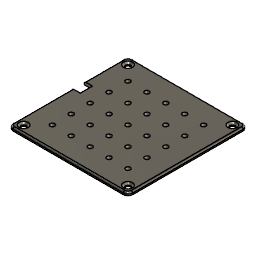
Box ESP32+CC1101 (Autodesk Fusion 360 design; units mm, degrees)
Autodesk Fusion 360 part; units mm, degrees
sketch "Base" plane through (0, 0, 0) normal (0, 0, 1) x (1, 0, 0)
  line L0 (-80.1103, 32.3186) -> (-1.1103, 32.3186)
  line L1 (-1.1103, 32.3186) -> (-1.1103, 111.3186)
  line L2 (-1.1103, 111.3186) -> (-80.1103, 111.3186)
  line L3 (-80.1103, 111.3186) -> (-80.1103, 32.3186)
  line L4 (-78.1103, 34.3186) -> (-3.1103, 34.3186)
  line L5 (-3.1103, 34.3186) -> (-3.1103, 109.3186)
  line L6 (-3.1103, 109.3186) -> (-78.1103, 109.3186)
  line L7 (-78.1103, 109.3186) -> (-78.1103, 34.3186)
  circle A0 centre (-75.1103, 106.3186) radius 5
  circle A1 centre (-6.1103, 106.3186) radius 5
  circle A2 centre (-6.1103, 37.3186) radius 5
  circle A3 centre (-75.1103, 37.3186) radius 5
  circle A4 centre (-70.6103, 106.3186) radius 2.5
  circle A5 centre (-10.6103, 106.3186) radius 2.5
  circle A6 centre (-70.6103, 48.3186) radius 2.5
  circle A7 centre (-10.6103, 48.3186) radius 2.5
  line L8 (-40.6103, 111.3186) -> (-40.6103, 44.5511) construction
  point P0 (-6.1103, 106.3186)
  point P1 (-75.1103, 106.3186)
  point P2 (-75.1103, 37.3186)
  point P3 (-6.1103, 37.3186)
  point P4 (-70.6103, 106.3186)
  point P5 (-10.6103, 106.3186)
  point P6 (-70.6103, 48.3186)
  point P7 (-10.6103, 48.3186)
  dimension "d206" = 79
  dimension "d207" = 79
  dimension "d209" = 5
  dimension "d211" = 5
  dimension "d212" = 5
  dimension "d213" = 5
  dimension "d272" = 60
  dimension "d273" = 7.5
  dimension "d276" = 3
  dimension "d278" = 60
  dimension "d279" = 7.5
  dimension "d280" = 58
  dimension "d281" = 5
  dimension "d282" = 5
  dimension "d283" = 5
  dimension "d284" = 5
  constraint horizontal L0
  constraint vertical L1
  constraint horizontal L2
  constraint vertical L3
  constraint tangent L2 A0
  constraint tangent L3 A0
  constraint tangent L2 A1
  constraint tangent L1 A1
  constraint tangent L1 A2
  constraint tangent L0 A2
  constraint tangent L3 A3
  constraint tangent L0 A3
  constraint coincident P0 A1.centre
  constraint coincident P1 A0.centre
  constraint coincident P2 A3.centre
  constraint coincident P3 A2.centre
  constraint coincident P4 A4.centre
  constraint coincident P5 A5.centre
  constraint coincident P6 A6.centre
  constraint coincident P7 A7.centre
  constraint midpoint L2 L8.start
  constraint perpendicular L6 L8
  measures "d206" distance of L0.start L0.end
  measures "d207" distance of L0.start L2.end
  measures "d209" radius of A0
  measures "d211" radius of A1
  measures "d212" radius of A2
  measures "d213" radius of A3
  measures "d272" distance of P4 P5
  measures "d273" distance of L7 P4
  measures "d276" distance of L6 P4
  measures "d278" distance of P6 P7
  measures "d279" distance of L7 P6
  measures "d280" distance of P4 P6
  measures "d281" diameter of A4
  measures "d282" diameter of A5
  measures "d283" diameter of A6
  measures "d284" diameter of A7
extrude "Extrude3" add sketch "Base" along normal blind 52 contours L0 L3 A3 | L0 L4 A2 A3 | L4 L7 A3 | L3 L7 A0 A3 | L0 L1 A2 | L4 L5 A2 | L4 L7 A3 | L2 L3 A0 | L6 L7 A0 | L4 L5 A2 | L1 L5 A1 A2 | L2 L6 A0 A1 | L6 L7 A0 A4 | L1 L2 A1 | L5 L6 A1 | A0 A4 | L5 L6 A1 A5 | A1 A5 picked at (-71.1053, 106.7133) picked at (-10.101, 106.3186) makes body 1
extrude "Extrude4" add sketch "Base" along normal blind 2 contours L4 L5 L6 L7 A0 A1 A2 A3 A4 A5 | A0 A4 | A1 A5 | A6 | A7 picked at (-69.4945, 106.7801) picked at (-11.7677, 106.3186) bodies 1
fillet "Fillet1" radius 3 4 edges at (-80.1103, 32.3186, 26) (-1.1103, 32.3186, 26) (-1.1103, 111.3186, 26) (-80.1103, 111.3186, 26) on bodies 1
sketch "Lid" plane through (0, 0, 52) normal (0, 0, 1) x (-1, 0, 0)
  arc A0 (77.1103, -111.3186) -> (80.1103, -108.3186) centre (77.1103, -108.3186) ccw
  line L0 (80.1103, -108.3186) -> (80.1103, -35.3186)
  arc A1 (80.1103, -35.3186) -> (77.1103, -32.3186) centre (77.1103, -35.3186) ccw
  line L1 (77.1103, -32.3186) -> (4.1103, -32.3186)
  arc A2 (4.1103, -32.3186) -> (1.1103, -35.3186) centre (4.1103, -35.3186) ccw
  line L2 (1.1103, -35.3186) -> (1.1103, -108.3186)
  arc A3 (1.1103, -108.3186) -> (4.1103, -111.3186) centre (4.1103, -108.3186) ccw
  line L3 (4.1103, -111.3186) -> (77.1103, -111.3186)
  line L4 (3.1103, -102.3186) -> (3.1103, -41.3186)
  arc A4 (3.1103, -41.3186) -> (10.1103, -34.3186) centre (6.1103, -37.3186) ccw
  line L5 (10.1103, -34.3186) -> (71.1103, -34.3186)
  arc A5 (71.1103, -34.3186) -> (78.1103, -41.3186) centre (75.1103, -37.3186) ccw
  line L6 (78.1103, -41.3186) -> (78.1103, -102.3186)
  arc A6 (78.1103, -102.3186) -> (71.1103, -109.3186) centre (75.1103, -106.3186) ccw
  line L7 (71.1103, -109.3186) -> (10.1103, -109.3186)
  arc A7 (10.1103, -109.3186) -> (3.1103, -102.3186) centre (6.1103, -106.3186) ccw
  line L8 (77.1103, -32.3186) -> (4.1103, -32.3186)
  line L9 (77.1103, -42.9754) -> (77.1103, -100.6617)
  arc A8 (77.1103, -100.6617) -> (69.4534, -108.3186) centre (75.1103, -106.3186) ccw
  line L10 (69.4534, -108.3186) -> (11.7671, -108.3186)
  arc A9 (11.7671, -108.3186) -> (4.1103, -100.6617) centre (6.1103, -106.3186) ccw
  line L11 (4.1103, -100.6617) -> (4.1103, -42.9754)
  arc A10 (4.1103, -42.9754) -> (11.7671, -35.3186) centre (6.1103, -37.3186) ccw
  line L12 (11.7671, -35.3186) -> (69.4534, -35.3186)
  arc A11 (69.4534, -35.3186) -> (77.1103, -42.9754) centre (75.1103, -37.3186) ccw
  circle A12 centre (65.6103, -46.8186) radius 1.5
  line L13 (80.1103, -82.3186) -> (74.6103, -82.3186)
  line L14 (74.6103, -82.3186) -> (74.6103, -74.3186)
  line L15 (74.6103, -74.3186) -> (80.1103, -74.3186)
  line L16 (80.1103, -74.3186) -> (80.1103, -82.3186)
  line L17 (78.1103, -70.5686) -> (75.1103, -70.5686)
  line L18 (75.1103, -70.5686) -> (75.1103, -72.5686)
  line L19 (75.1103, -72.5686) -> (74.1103, -72.5686)
  line L20 (74.1103, -72.5686) -> (74.1103, -69.5686)
  line L21 (74.1103, -69.5686) -> (78.1103, -69.5686)
  line L22 (74.6103, -78.3186) -> (92.1039, -78.3186)
  line L23 (78.1103, -69.5686) -> (78.1103, -70.5686)
  line L24 (78.1103, -86.0686) -> (75.1103, -86.0686)
  line L25 (75.1103, -86.0686) -> (75.1103, -84.0686)
  line L26 (75.1103, -84.0686) -> (74.1103, -84.0686)
  line L27 (74.1103, -84.0686) -> (74.1103, -87.0686)
  line L28 (74.1103, -87.0686) -> (78.1103, -87.0686)
  line L29 (78.1103, -87.0686) -> (78.1103, -86.0686)
  point P0 (6.1103, -106.3186)
  point P1 (6.1103, -37.3186)
  point P2 (75.1103, -37.3186)
  point P3 (75.1103, -106.3186)
  point P4 (6.1103, -37.3186)
  point P5 (6.1103, -106.3186)
  point P6 (75.1103, -106.3186)
  point P7 (75.1103, -37.3186)
  dimension "d226" = 1
  dimension "d300" = 3
  dimension "d301" = 12.5
  dimension "d302" = 12.5
  dimension "d331" = 5.5
  dimension "d332" = 8
  dimension "d338" = 27
  dimension "d343" = 3
  dimension "d344" = 2
  dimension "d345" = 1
  dimension "d346" = 3
  dimension "d347" = 3.75
  constraint coincident P4 P1
  constraint coincident P5 P0
  constraint coincident P6 P3
  constraint coincident P7 P2
  constraint horizontal L13
  constraint vertical L14
  constraint horizontal L15
  constraint vertical L16
  constraint coincident L0 L13.start
  constraint coincident L6 L17.start
  constraint perpendicular L9 L17
  constraint perpendicular L17 L18
  constraint perpendicular L18 L19
  constraint perpendicular L19 L20
  constraint coincident L6 L21.end
  constraint perpendicular L6 L21
  constraint midpoint L14 L22.start
  constraint perpendicular L14 L22
  constraint symmetric L17.start L22 L24.start
  constraint symmetric L17.end L22 L24.end
  constraint symmetric L18.end L22 L25.end
  constraint symmetric L19.end L22 L26.end
  constraint symmetric L20.end L22 L27.end
  constraint symmetric L21.end L22 L28.end
  measures "d300" diameter of A12
  measures "d301" distance of L6 A12.centre
  measures "d302" distance of L5 A12.centre
  measures "d331" distance of L13.start L13.end
  measures "d332" distance of L13.start L15.end
  measures "d338" distance of L7 L13
  measures "d343" distance of L17.start L17.end
  measures "d344" distance of L17.end L18.end
  measures "d345" distance of L18.end L19.end
  measures "d346" distance of L19.end L20.end
  measures "d347" distance of L15 L17
hole "Hole1" at (-6.1103, 106.3186, 52) at (-6.1103, 37.3186, 52) at (-75.1103, 37.3186, 52) at (-75.1103, 106.3186, 52) direction (0, 0, -1) diameter 4 depth 7 tip angle 118 bodies 1
extrude "Extrude6" add sketch "Lid" against normal blind 1.5 separate body contours L9 L13 L14 L22 | L9 A8 L10 A9 L11 A10 L12 A11 L13 L14 L15 L17 L18 L19 L20 L21 L24 L25 L26 L27 L28 | L9 L14 L15 L22 | L9 L24 L25 L26 L27 L28 | L9 L17 L18 L19 L20 L21 | A12 makes body 2
extrude "Extrude7" add sketch "Lid" along normal blind 2 separate body contours A0 L0 A1 L1 A2 L2 A3 L3 L4 A4 L5 A5 L6 A6 L7 A7 L8 L13 L15 L23 L29 | L0 L6 L13 L16 L22 | L0 L6 L15 L16 L22 | L6 L9 L13 L22 | L6 L9 L13 L24 | L6 L9 L15 L22 | L6 L9 L24 L28 L29 | L9 L13 L14 L22 | L9 A8 L10 A9 L11 A10 L12 A11 L13 L14 L15 L17 L18 L19 L20 L21 L24 L25 L26 L27 L28 | L6 L9 L15 L17 | L9 L14 L15 L22 | L4 A4 L5 A5 L6 A6 L7 A7 L9 A8 L10 A9 L11 A10 L12 A11 L21 L28 | L9 L24 L25 L26 L27 L28 | L6 L9 L17 L21 L23 | L9 L17 L18 L19 L20 L21 | A12 makes body 3
combine "Combine1" operation add target body 2 tool bodies 3
sketch "Screwholes" plane through (0, 0, 54) normal (0, 0, 1) x (-1, 0, 0)
  line L0 (77.1103, -32.3186) -> (4.1103, -32.3186)
  arc A0 (4.1103, -32.3186) -> (1.1103, -35.3186) centre (4.1103, -35.3186) ccw
  line L1 (1.1103, -35.3186) -> (1.1103, -108.3186)
  arc A1 (1.1103, -108.3186) -> (4.1103, -111.3186) centre (4.1103, -108.3186) ccw
  line L2 (4.1103, -111.3186) -> (77.1103, -111.3186)
  arc A2 (77.1103, -111.3186) -> (80.1103, -108.3186) centre (77.1103, -108.3186) ccw
  line L3 (80.1103, -108.3186) -> (80.1103, -35.3186)
  arc A3 (80.1103, -35.3186) -> (77.1103, -32.3186) centre (77.1103, -35.3186) ccw
  line L4 (3.1103, -102.3186) -> (3.1103, -41.3186)
  line L5 (10.1103, -34.3186) -> (71.1103, -34.3186)
  point P0 (75.1103, -106.3186)
  point P1 (6.1103, -106.3186)
  point P2 (6.1103, -37.3186)
  point P3 (75.1103, -37.3186)
  point P4 (75.1103, -106.3186)
  point P5 (75.1103, -37.3186)
  point P6 (6.1103, -37.3186)
  point P7 (6.1103, -106.3186)
  point P8 (15.6103, -46.8186)
  point P9 (28.1103, -46.8186)
  point P10 (40.6103, -46.8186)
  point P11 (15.6103, -59.3186)
  point P12 (28.1103, -59.3186)
  point P13 (40.6103, -59.3186)
  point P14 (15.6103, -71.8186)
  point P15 (28.1103, -71.8186)
  point P16 (40.6103, -71.8186)
  point P17 (15.6103, -84.3186)
  point P18 (28.1103, -84.3186)
  point P19 (40.6103, -84.3186)
  point P20 (15.6103, -96.8186)
  point P21 (28.1103, -96.8186)
  point P22 (40.6103, -96.8186)
  point P23 (53.1103, -46.8186)
  point P24 (65.6103, -46.8186)
  point P25 (53.1103, -59.3186)
  point P26 (65.6103, -59.3186)
  point P27 (53.1103, -71.8186)
  point P28 (65.6103, -71.8186)
  point P29 (53.1103, -84.3186)
  point P30 (65.6103, -84.3186)
  point P31 (53.1103, -96.8186)
  point P32 (65.6103, -96.8186)
  dimension "d263" = 12.5
  dimension "d264" = 12.5
  dimension "d267" = 50
  dimension "d268" = -50
  constraint coincident P4 P0
  constraint coincident P5 P3
  constraint coincident P6 P2
  constraint coincident P7 P1
  measures "d263" distance of P8 L4
  measures "d264" distance of P8 L5
hole "Hole2" at (-75.1103, 106.3186, 54) at (-6.1103, 106.3186, 54) at (-75.1103, 37.3186, 54) at (-6.1103, 37.3186, 54) direction (0, 0, -1) diameter 3.5 depth 3 tip angle 118 countersink diameter 6 countersink angle 90 bodies 2
fillet "Fillet2" radius 1 8 edges at (-1.1103, 71.8186, 54) (-1.989, 110.4399, 54) (-40.6103, 111.3186, 54) (-79.2316, 110.4399, 54) (-80.1103, 71.8186, 54) (-79.2316, 33.1973, 54) (-40.6103, 32.3186, 54) (-1.989, 33.1973, 54) on bodies 2
fillet "Fillet3" radius 0.5 8 edges at (-70.8676, 102.0759, 50.5) (-40.6103, 108.3186, 50.5) (-77.1103, 71.8186, 50.5) (-70.8676, 41.5612, 50.5) (-40.6103, 35.3186, 50.5) (-10.3529, 41.5612, 50.5) (-4.1103, 71.8186, 50.5) (-10.3529, 102.0759, 50.5) on bodies 2
sketch "Vent Slits" plane through (-80.1103, 0, 0) normal (-1, 0, 0) x (0, -1, 0)
  line L0 (-108.3186, 52) -> (-108.3186, 0)
  line L1 (-108.3186, 0) -> (-35.3186, 0)
  line L2 (-35.3186, 0) -> (-35.3186, 52)
  line L3 (-35.3186, 52) -> (-108.3186, 52)
  line L4 (-91.5686, 41) -> (-91.5686, 33.5)
  line L5 (-89.5686, 33.5) -> (-89.5686, 41)
  line L6 (-108.3186, 52) -> (-35.3186, 52)
  line L7 (-108.3186, 0) -> (-108.3186, 52)
  arc A0 (-90.5686, 42) -> (-91.5686, 41) centre (-90.5686, 41) ccw
  arc A1 (-89.5686, 41) -> (-90.5686, 42) centre (-90.5686, 41) ccw
  arc A2 (-91.5686, 33.5) -> (-90.5686, 32.5) centre (-90.5686, 33.5) ccw
  arc A3 (-90.5686, 32.5) -> (-89.5686, 33.5) centre (-90.5686, 33.5) ccw
  point P0 (-89.5686, 42)
  point P1 (-91.5686, 42)
  point P2 (-89.5686, 32)
  dimension "d240" = 2
  dimension "d241" = 10
  dimension "d243" = 16.75
  dimension "d244" = 1
  dimension "d245" = 1
  dimension "d246" = 1
  dimension "d247" = 1
  dimension "d254" = 10
  constraint vertical L4
  constraint vertical L5
  constraint coincident P1 L4
  constraint tangent L4 A0
  constraint coincident P0 L5
  constraint tangent L5 A1
  constraint coincident A0.start A1.end
  constraint tangent L4 A2
  constraint coincident P2 L5
  constraint tangent L5 A3
  constraint coincident A2.end A3.start
  measures "d240" distance of P0 P1
  measures "d241" distance of P0 P2
  measures "d243" distance of L4 L7
  measures "d244" radius of A0
  measures "d245" radius of A1
  measures "d246" radius of A2
  measures "d247" radius of A3
  measures "d254" distance of L3 A0.start
extrude "Extrude8" cut sketch "Vent Slits" against normal blind 3 contours L4 L5 A0 A1 A2 A3 bodies 1
pattern_linear "R-Pattern1" count 2 spacing 20 along (0, 0, -1) of "Extrude8"
pattern_linear "R-Pattern2" count 3 spacing 18.75 along (0, -1, 0) of "Extrude8", "R-Pattern1"
extrude "Extrude9" add sketch "Base" along normal blind 7 separate body contours A0 A4 | A0 A4 | A1 A5 | A1 A5 | A6 | A7 makes body 4 at (-12.914, 105.3475, 2.3333) makes body 5 at (-68.1134, 48.194, 4.6667) makes body 6 at (-68.3066, 107.2897, 4.6667) makes body 7 at (-8.1134, 48.194, 4.6667)
sketch "DistHolderTop" plane through (0, 0, 7) normal (0, 0, 1) x (-1, 0, 0)
  circle A0 centre (40.6103, -121.3186) radius 2.5
  circle A1 centre (70.6103, -106.3186) radius 2.5
  line L0 (4.1103, -111.3186) -> (77.1103, -111.3186)
  circle A2 centre (75.1103, -37.3186) radius 2
  circle A3 centre (6.1103, -106.3186) radius 2
  circle A4 centre (6.1103, -37.3186) radius 2
  circle A5 centre (75.1103, -106.3186) radius 2
  arc A6 (77.1103, -111.3186) -> (80.1103, -108.3186) centre (77.1103, -108.3186) ccw
  line L1 (80.1103, -108.3186) -> (80.1103, -35.3186)
  arc A7 (80.1103, -35.3186) -> (77.1103, -32.3186) centre (77.1103, -35.3186) ccw
  line L2 (77.1103, -32.3186) -> (4.1103, -32.3186)
  arc A8 (4.1103, -32.3186) -> (1.1103, -35.3186) centre (4.1103, -35.3186) ccw
  line L3 (1.1103, -35.3186) -> (1.1103, -108.3186)
  arc A9 (1.1103, -108.3186) -> (4.1103, -111.3186) centre (4.1103, -108.3186) ccw
  line L4 (4.1103, -111.3186) -> (77.1103, -111.3186)
  line L5 (3.1103, -102.3186) -> (3.1103, -41.3186)
  arc A10 (3.1103, -41.3186) -> (10.1103, -34.3186) centre (6.1103, -37.3186) ccw
  line L6 (10.1103, -34.3186) -> (71.1103, -34.3186)
  arc A11 (71.1103, -34.3186) -> (78.1103, -41.3186) centre (75.1103, -37.3186) ccw
  line L7 (78.1103, -41.3186) -> (78.1103, -102.3186)
  arc A12 (78.1103, -102.3186) -> (71.1103, -109.3186) centre (75.1103, -106.3186) ccw
  line L8 (71.1103, -109.3186) -> (10.1103, -109.3186)
  arc A13 (10.1103, -109.3186) -> (3.1103, -102.3186) centre (6.1103, -106.3186) ccw
  line L9 (78.1103, -108.3186) -> (78.1103, -35.3186)
  arc A14 (78.1103, -35.3186) -> (77.1103, -34.3186) centre (77.1103, -35.3186) ccw
  line L10 (77.1103, -34.3186) -> (4.1103, -34.3186)
  arc A15 (4.1103, -34.3186) -> (3.1103, -35.3186) centre (4.1103, -35.3186) ccw
  line L11 (3.1103, -35.3186) -> (3.1103, -108.3186)
  arc A16 (3.1103, -108.3186) -> (4.1103, -109.3186) centre (4.1103, -108.3186) ccw
  line L12 (4.1103, -109.3186) -> (77.1103, -109.3186)
  arc A17 (77.1103, -109.3186) -> (78.1103, -108.3186) centre (77.1103, -108.3186) ccw
  point P0 (40.6103, -121.3186)
  point P1 (13.1103, -121.3186)
  point P2 (40.6103, -77.3186)
  point P3 (13.1103, -77.3186)
sketch "USB Hole" plane through (0, 111.3186, 0) normal (0, 1, 0) x (-1, 0, 0)
  line L0 (77.1103, 0) -> (77.1103, 52)
  line L1 (77.1103, 52) -> (4.1103, 52)
  line L2 (4.1103, 52) -> (4.1103, 0)
  line L3 (4.1103, 0) -> (77.1103, 0)
  line L4 (40.6103, 0) -> (40.6103, 68.2692) construction
  line L5 (35.6103, 26) -> (45.6103, 26)
  line L6 (46.6103, 25) -> (46.6103, 19)
  line L7 (45.6103, 18) -> (35.6103, 18)
  line L8 (34.6103, 19) -> (34.6103, 25)
  line L9 (80.1103, 0) -> (1.1103, 0)
  arc A0 (46.6103, 25) -> (45.6103, 26) centre (45.6103, 25) ccw
  arc A1 (35.6103, 26) -> (34.6103, 25) centre (35.6103, 25) ccw
  arc A2 (34.6103, 19) -> (35.6103, 18) centre (35.6103, 19) ccw
  arc A3 (45.6103, 18) -> (46.6103, 19) centre (45.6103, 19) ccw
  line L10 (44.6103, 42) -> (36.6103, 42)
  line L11 (36.6103, 42) -> (36.6103, 34)
  line L12 (36.6103, 34) -> (44.6103, 34)
  line L13 (44.6103, 34) -> (44.6103, 42)
  point P0 (34.6103, 26)
  point P1 (46.6103, 26)
  point P2 (34.6103, 18)
  dimension "d290" = 12
  dimension "d291" = 8
  dimension "d293" = 6
  dimension "d294" = 18
  dimension "d295" = 1
  dimension "d362" = 8
  dimension "d363" = 8
  dimension "d365" = 8
  dimension "d366" = 4
  constraint midpoint L3 L4.start
  constraint perpendicular L1 L4
  constraint horizontal L5
  constraint vertical L6
  constraint horizontal L7
  constraint vertical L8
  constraint coincident P1 L6
  constraint coincident P1 L5
  constraint tangent L6 A0
  constraint tangent L5 A0
  constraint coincident P0 L5
  constraint coincident P0 L8
  constraint tangent L5 A1
  constraint tangent L8 A1
  constraint equal A0 A1
  constraint coincident P2 L8
  constraint coincident P2 L7
  constraint tangent L8 A2
  constraint tangent L7 A2
  constraint equal A0 A2
  constraint tangent L7 A3
  constraint tangent L6 A3
  constraint equal A0 A3
  constraint horizontal L10
  constraint vertical L11
  constraint horizontal L12
  constraint vertical L13
  measures "d290" distance of P0 P1
  measures "d291" distance of P0 P2
  measures "d293" distance of L4 L6
  measures "d294" distance of L7 L9
  measures "d295" radius of A0
  measures "d362" distance of L10.start L10.end
  measures "d363" distance of L10.start L12.end
  measures "d365" distance of L5 L12
  measures "d366" distance of L4 L11
combine "Combine2" operation add target body 1 tool bodies 4 5 6 7
extrude "Extrude10" cut sketch "USB Hole" against normal blind 3 contours L5 L6 L7 L8 A0 A1 A2 A3 bodies 1
fillet "Fillet4" radius 1 8 edges at (-46.3174, 111.3186, 25.7071) (-46.6103, 111.3186, 22) (-46.3174, 111.3186, 18.2929) (-40.6103, 111.3186, 18) (-34.9032, 111.3186, 18.2929) (-34.6103, 111.3186, 22) (-34.9032, 111.3186, 25.7071) (-40.6103, 111.3186, 26) on bodies 1
extrude "Extrude11" cut sketch "Lid" along normal blind -1.5 and the other way blind -2 contours A12 bodies 2
pattern_linear "R-Pattern3" count 5 spacing 12.5 along (1, 0, 0) count 5 spacing 12.5 along (0, 1, 0) of 1 faces at (-66.9276, 46.1012, 51.6667) on bodies 2
extrude "Extrude12" cut sketch "DistHolderTop" along normal blind 30 contours A1 A12 | A1 A12 L9 L12 A17 | A5 | A13 L11 A16 L12 | A3 picked at (71.1196, -106.3186) bodies 1
extrude "Extrude13" cut sketch "DistHolderTop" along normal blind 0.0001 contours A11 L9 A14 L10 | A10 L10 A15 L11 | A2 | A4 bodies 1
ref_plane "WorkPlane1" through (-72.8978, 105.1433, 7) normal (0, 0, 1) x (1, 0, 0)
sketch "Mnt_Holes" plane through (0, 0, 7) normal (0, 0, 1) x (1, 0, 0)
  point P0 (-10.6103, 106.3186)
  point P1 (-70.6103, 106.3186)
  point P2 (-70.6103, 48.3186)
  point P3 (-10.6103, 48.3186)
hole "Hole6" at (-70.6103, 106.3186, 7) at (-10.6103, 106.3186, 7) at (-10.6103, 48.3186, 7) at (-70.6103, 48.3186, 7) direction (0, 0, -1) diameter 2 depth 4 tip angle 180 bodies 1
extrude "Extrude14" cut sketch "Lid" along normal blind 2 and the other way blind 1.5 contours L0 L6 L13 L16 L22 | L0 L6 L15 L16 L22 | L6 L9 L13 L22 | L6 L9 L15 L22 | L9 L13 L14 L22 | L9 L14 L15 L22 bodies 2
ref_plane "WorkPlane2" through (-40.6103, 71.8186, 49.5) normal (0, 0, -1) x (1, 0, 0)
sketch "Rx Holder" plane through (0, 0, 49.5) normal (0, 0, -1) x (-1, 0, 0)
  line L0 (78.1103, 70.5686) -> (75.1103, 70.5686)
  line L1 (75.1103, 70.5686) -> (75.1103, 72.5686)
  line L2 (75.1103, 72.5686) -> (74.1103, 72.5686)
  line L3 (74.1103, 72.5686) -> (74.1103, 69.5686)
  line L4 (74.1103, 69.5686) -> (78.1103, 69.5686)
  line L5 (78.1103, 69.5686) -> (78.1103, 70.5686)
  line L6 (75.1103, 84.0686) -> (74.1103, 84.0686)
  line L7 (74.1103, 84.0686) -> (74.1103, 87.0686)
  line L8 (74.1103, 87.0686) -> (78.1103, 87.0686)
  line L9 (78.1103, 87.0686) -> (78.1103, 86.0686)
  line L10 (75.1103, 86.0686) -> (75.1103, 84.0686)
  line L11 (78.1103, 86.0686) -> (75.1103, 86.0686)
extrude "Extrude16" add sketch "Rx Holder" along normal blind 30 separate body makes body 8 at (-75.4436, 69.5686, 39.5) makes body 9 at (-75.4436, 87.0686, 39.5)
fillet "Fillet5" radius 1 4 edges at (-76.6103, 70.5686, 49.5) (-75.1103, 71.5686, 49.5) (-76.6103, 86.0686, 49.5) (-75.1103, 85.0686, 49.5) on bodies 8 9
sketch "RX Holder 2" plane through (0, 69.5686, 0) normal (0, -1, 0) x (1, 0, 0)
  line L0 (-74.1103, 49.5) -> (-78.1103, 49.5)
  line L1 (-78.1103, 49.5) -> (-78.1103, 19.5)
  line L2 (-74.1103, 19.5) -> (-74.1103, 49.5)
  line L3 (-78.1103, 19.5) -> (-78.1103, 16)
  line L4 (-78.1103, 16) -> (-74.1103, 19.5)
  line L5 (-78.1103, 19.5) -> (-74.1103, 19.5)
  dimension "d359" = 3.5
  constraint coincident L1.end L3.start
  constraint parallel L1 L3
  constraint coincident L2.start L4.end
  measures "d359" distance of L1.end L3.end
extrude "Extrude19" add sketch "RX Holder 2" against normal blind 17.5 contours L3 L4 L5 bodies 1 8 9
extrude "Extrude20" cut sketch "USB Hole" against normal blind 2 contours L10 L11 L12 L13 bodies 1
fillet "Fillet6" radius 0.3333 4 edges at (-36.6103, 111.3186, 38) (-40.6103, 111.3186, 42) (-44.6103, 111.3186, 38) (-40.6103, 111.3186, 34) on bodies 1
fillet "Fillet7" radius 0.6667 4 edges at (-40.6103, 109.3186, 34) (-44.6103, 109.3186, 38) (-40.6103, 109.3186, 42) (-36.6103, 109.3186, 38) on bodies 1
sketch "Sketch24" plane through (-80.1103, 0, 0) normal (-1, 0, 0) x (0, -1, 0)
  line L0 (-52.0686, 21) -> (-52.0686, 13.5)
  arc A0 (-54.0686, 13.5) -> (-52.0686, 13.5) centre (-53.0686, 13.5) ccw
  line L1 (-54.0686, 13.5) -> (-54.0686, 21)
  arc A1 (-52.0686, 21) -> (-54.0686, 21) centre (-53.0686, 21) ccw
  line L2 (-52.0686, 41) -> (-52.0686, 33.5)
  arc A2 (-54.0686, 33.5) -> (-52.0686, 33.5) centre (-53.0686, 33.5) ccw
  line L3 (-54.0686, 33.5) -> (-54.0686, 41)
  arc A3 (-52.0686, 41) -> (-54.0686, 41) centre (-53.0686, 41) ccw
  line L4 (-70.8186, 21) -> (-70.8186, 13.5)
  arc A4 (-72.8186, 13.5) -> (-70.8186, 13.5) centre (-71.8186, 13.5) ccw
  line L5 (-72.8186, 13.5) -> (-72.8186, 21)
  arc A5 (-70.8186, 21) -> (-72.8186, 21) centre (-71.8186, 21) ccw
  line L6 (-70.8186, 41) -> (-70.8186, 33.5)
  arc A6 (-72.8186, 33.5) -> (-70.8186, 33.5) centre (-71.8186, 33.5) ccw
  line L7 (-72.8186, 33.5) -> (-72.8186, 41)
  arc A7 (-70.8186, 41) -> (-72.8186, 41) centre (-71.8186, 41) ccw
  line L8 (-89.5686, 21) -> (-89.5686, 13.5)
  arc A8 (-91.5686, 13.5) -> (-89.5686, 13.5) centre (-90.5686, 13.5) ccw
  line L9 (-91.5686, 13.5) -> (-91.5686, 21)
  arc A9 (-89.5686, 21) -> (-91.5686, 21) centre (-90.5686, 21) ccw
  line L10 (-89.5686, 41) -> (-89.5686, 33.5)
  arc A10 (-91.5686, 33.5) -> (-89.5686, 33.5) centre (-90.5686, 33.5) ccw
  line L11 (-91.5686, 33.5) -> (-91.5686, 41)
  arc A11 (-89.5686, 41) -> (-91.5686, 41) centre (-90.5686, 41) ccw
  line L12 (-108.3186, 52) -> (-108.3186, 0)
  line L13 (-108.3186, 0) -> (-35.3186, 0)
  line L14 (-35.3186, 0) -> (-35.3186, 52)
  line L15 (-35.3186, 52) -> (-108.3186, 52)
  line L16 (-82.2518, 52) -> (-74.2518, 52)
  line L17 (-74.2518, 52) -> (-74.2518, 50.5)
  line L18 (-74.2518, 50.5) -> (-82.2518, 50.5)
  line L19 (-82.2518, 50.5) -> (-82.2518, 52)
  dimension "d373" = 8
  dimension "d374" = 1.5
  constraint horizontal L16
  constraint vertical L17
  constraint horizontal L18
  constraint vertical L19
  constraint coincident L15 L16.start
  measures "d373" distance of L16.start L16.end
  measures "d374" distance of L16.start L18.end
extrude "Extrude21" cut sketch "Sketch24" against normal blind 2 contours L15 L16 L17 L18 L19 bodies 1
hidden bodies 1
equation "bx_inner_width = 75 mm"
equation "bx_inner_length = 75 mm"
equation "bx_inner_depth = 50 mm" comment "Box dimensions"
equation "bx_wall_strength = 2 mm"
equation "lid_heigth = 2 mm" comment "Lid parameter"
equation "lid_gap = 1 mm" comment "Distance of walls to inner lid part"
equation "lid_overlap = 1.5 mm" comment "Depth of lid part reaching into box"
equation "vent_slit_h = 10 mm"
equation "vent_slit_w = 2 mm"
equation "vent_slit_count = 3" comment "Parameter for ventilation slits (box, one side). Also includes # of rows"
equation "vent_holes_lng = 5"
equation "vent_holes_w = 5"
equation "vent_holes_dia = 3 mm" comment "Ventilation holes (lid) parameter"
equation "vent_slit_rows = 2"
equation "xx_vent_slit_dist_vert = ( bx_inner_depth - vent_slit_h * vent_slit_rows ) / ( vent_slit_rows + 1 )" comment "Helper - do not change"
equation "xx_vents_slit_dist_hor = ( bx_inner_length + 2 * ( bx_wall_strength - x_fillet_edge ) - ( vent_slit_w * vent_slit_count ) ) / ( vent_slit_count + 1 )" comment "Helper - do not change"
equation "d206 = bx_inner_width + 2 * bx_wall_strength"
equation "d207 = bx_inner_length + 2 * bx_wall_strength"
equation "d208 = -bx_wall_strength"
equation "d209 = pillar_dia"
equation "pillar_dia = 5 mm" comment "Diameter of box edge pillars"
equation "d211 = pillar_dia"
equation "d212 = pillar_dia"
equation "d213 = pillar_dia"
equation "d214 = bx_inner_depth + bx_wall_strength"
equation "d216 = bx_wall_strength"
equation "x_fillet_edge = 3 mm" comment "Large fillet dimension"
equation "d220 = x_fillet_edge"
equation "d222 = pillar_holes"
equation "d226 = lid_gap"
equation "d227 = -lid_overlap"
equation "d229 = lid_heigth"
equation "d231 = lid_heigth + 1 mm"
equation "d237 = x_fillet_small"
equation "d239 = x_fillet_small / 2"
equation "d240 = vent_slit_w"
equation "d241 = vent_slit_h"
equation "d243 = xx_vents_slit_dist_hor"
equation "d244 = vent_slit_w / 2"
equation "d245 = vent_slit_w / 2"
equation "d246 = vent_slit_w / 2"
equation "d247 = vent_slit_w / 2"
equation "d248 = -bx_wall_strength - 1 mm"
equation "d250 = vent_slit_rows"
equation "d252 = ( vent_slit_h + xx_vent_slit_dist_vert ) * ( vent_slit_rows - 1 )"
equation "d254 = xx_vent_slit_dist_vert"
equation "d255 = vent_slit_count"
equation "d257 = ( vent_slit_w + xx_vents_slit_dist_hor ) * ( vent_slit_count - 1 )"
equation "x_fillet_small = 1 mm" comment "Small fillet dimension"
equation "xx_vent_hole_dist_l = bx_inner_length / ( vent_holes_lng + 1 )" comment "Helper - do not change"
equation "xx_vent_hole_dist_w = bx_inner_width / ( vent_holes_w + 1 )" comment "Helper - do not change"
equation "d263 = xx_vent_hole_dist_w"
equation "d264 = xx_vent_hole_dist_l"
equation "d265 = vent_holes_w"
equation "d266 = vent_holes_lng"
equation "d267 = xx_vent_hole_dist_w * ( vent_holes_w - 1 )"
equation "d268 = -xx_vent_hole_dist_l * ( vent_holes_lng - 1 )"
equation "d272 = PCB_mnt_dist_w"
equation "d273 = ( bx_inner_width - PCB_mnt_dist_w ) / 2"
equation "PCB_mnt_dist_w = 60 mm" comment "Distance/width of PCB mounting holes"
equation "PCB_mnt_dist_l = 58 mm" comment "Distance/length of PCB mounting holes"
equation "d278 = PCB_mnt_dist_w"
equation "d279 = ( bx_inner_width - PCB_mnt_dist_w ) / 2"
equation "d280 = PCB_mnt_dist_l"
equation "d281 = PCB_mount_dia"
equation "d282 = PCB_mount_dia"
equation "d283 = PCB_mount_dia"
equation "d284 = PCB_mount_dia"
equation "d285 = PCB_mount_h + bx_wall_strength"
equation "d290 = USB_cutout_w"
equation "d291 = USB_cutout_h"
equation "USB_cutout_h = 8 mm" comment "Height of USB hole - 8mm for USB-C / smaller Micro USB"
equation "d293 = USB_cutout_w / 2"
equation "d294 = bx_wall_strength + PCB_mount_h + USB_cutout_vert_dist"
equation "d296 = -bx_wall_strength - 1 mm"
equation "d300 = vent_holes_dia"
equation "d301 = xx_vent_hole_dist_w"
equation "d302 = xx_vent_hole_dist_l"
equation "d303 = -lid_overlap"
equation "d305 = -lid_heigth"
equation "d307 = vent_holes_w"
equation "d308 = vent_holes_lng"
equation "d309 = xx_vent_hole_dist_w * ( vent_holes_w - 1 )"
equation "d310 = xx_vent_hole_dist_l * ( vent_holes_lng - 1 )"
equation "PCB_mount_h = 5 mm"
equation "PCB_mount_dia = 5 mm" comment "Parameter for PCB mounting pillars"
equation "PCB_mount_hole_dia = 2 mm"
equation "d317 = -bx_wall_strength"
equation "pillar_cutout_front_h = 30 mm" comment "Cutout of front pillars to accomodate PCB (if inner width - pillars smaller than PCD width)"
equation "pillar_cutout_back_h = 0.0001 mm" comment "Cutout of back pillars to accomodate PCB (if needed)"
equation "d320 = pillar_cutout_front_h"
equation "d322 = pillar_cutout_back_h"
equation "pillar_holes = 4 mm" comment "Holes for threaded heat inserts (e.g. 4mm) Use e.g  2.mm if just using screws"
equation "USB_cutout_vert_dist = 11 mm" comment "Vertical distance from PCB to USB"
equation "USB_cutout_w = 12 mm"
equation "d328 = PCB_mount_h - 1 mm"
equation "d329 = PCB_mount_hole_dia"
equation "d333 = lid_heigth"
equation "d335 = lid_overlap"
equation "d352 = x_fillet_small"
equation "d362 = led_cutout"
equation "d363 = led_cutout"
equation "led_cutout = 8 mm" comment "8mm with lens - 5mm direct chip"
equation "d366 = led_cutout / 2"
equation "d367 = -bx_wall_strength"
equation "d370 = bx_wall_strength / 3 / 2"
equation "d372 = bx_wall_strength / 3"
equation "d375 = -bx_wall_strength"
named bodies: "Box", "Lid"
